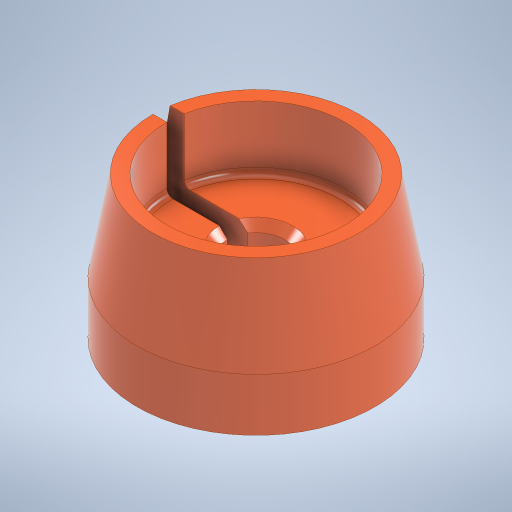
# Autodesk Inventor part: Ferula macho Fiber Op
Saved by Autodesk Inventor 2024.2 (Build 282272000, 272)
## iProperties
Created: 2025-06-04
Part Number: Ferula macho Fiber Op
Material: Phenolic Resin
Document SubType Name: Modeling
Designer: ja.restrepo1
Density: 1.38 g/cm^3
Appearance: Smooth - Light Orange
Author: ja.restrepo1
Autodesk Inventor part; units mm, degrees
ref_plane "YZ Plane" through (0, 0, 0) normal (1, 0, 0) x (0, 1, 0)
ref_plane "XZ Plane" through (0, 0, 0) normal (0, 1, 0) x (-1, 0, 0)
ref_plane "XY Plane" through (0, 0, 0) normal (0, 0, 1) x (1, 0, 0)
sketch "Sketch1" plane through (0, 0, 0) normal (0, 1, 0) x (-1, 0, 0)
  arc A0 (0.725, 0) -> (0.6047, -0.4) centre (0, 0) ccw
  arc A1 (2.25, 0) -> (2.2142, -0.4) centre (0, 0) ccw
  arc A2 (3, 0) -> (2.9732, -0.4) centre (0, 0) ccw
  line L0 (0.725, 0) -> (3, 0)
  arc A3 (2.9886, -0.2615) -> (3, 0) centre (0, 0) ccw construction
  arc A4 (2.2414, -0.1961) -> (2.25, 0) centre (0, 0) ccw construction
  arc A5 (0.7222, -0.0632) -> (0.725, 0) centre (0, 0) ccw construction
  line L1 (0.6047, -0.4) -> (2.9732, -0.4)
  arc A6 (0.6047, -0.4) -> (0.7222, -0.0632) centre (0, 0) ccw construction
  arc A7 (2.2142, -0.4) -> (2.2414, -0.1961) centre (0, 0) ccw construction
  point P0 (1.8625, 0)
  dimension "d0" = 1.45
  dimension "d1" = 4.5
  dimension "d2" = 6
  dimension "d15" = 0.4
  constraints: 18 point on circle, 8 centre point, 4 end point, 3 coincident, 2 horizontal, 2 point on line, 1 horizontal alignment, 1 midpoint
  measures "d0" diameter of A0
  measures "d1" diameter of A1
  measures "d2" diameter of A2
  measures "d15" distance between parallel lines of L1 L0
extrude "Extrusion1" add sketch "Sketch1" along normal blind 2
extrude "Extrusion2" add sketch "Sketch1" along normal blind 3.6 contours A1 L1 A2 L0
chamfer "Chamfer1" distance 0.4 angle 80 1 edges at (2.9933, 3.6, 0.2004) measured on face at (2.4944, 3.6, 0.167)
chamfer "Chamfer2" distance 0.2 angle 45 2 edges at (0.6943, 2, 0.2089) (0.6943, 0, 0.2089)
fillet "Fillet2" radius 0.15 1 edges at (2.241, 2, 0.2008)
body "Solid1"
